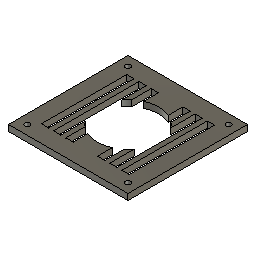
Back Plate (Autodesk Fusion 360 design; units mm, degrees)
part number: 2026-08-30-01-23-59-414
Autodesk Fusion 360 part; units mm, degrees
sketch "Sketch1" plane through (0, 0, 0) normal (0, 0, 1) x (1, 0, 0)
  line L0 (0, 0) -> (98, 0)
  line L1 (98, 0) -> (98, 98)
  line L2 (98, 98) -> (0, 98)
  line L3 (0, 98) -> (0, 0)
extrude "Extrude1" add sketch "Sketch1" along normal blind 5
sketch "Sketch2" plane through (0, 0, 0) normal (0, 0, 1) x (1, 0, 0)
  circle A0 centre (7.75, 7.75) radius 2.1
extrude "Extrude2" cut sketch "Sketch2" along normal blind 5
sketch "Sketch3" plane through (0, 0, 0) normal (0, 0, 1) x (1, 0, 0)
  circle A0 centre (7.75, 90.25) radius 2.1
extrude "Extrude3" cut sketch "Sketch3" along normal blind 5
sketch "Sketch4" plane through (0, 0, 0) normal (0, 0, 1) x (1, 0, 0)
  circle A0 centre (90.25, 7.75) radius 2.1
extrude "Extrude4" cut sketch "Sketch4" along normal blind 5
sketch "Sketch5" plane through (0, 0, 0) normal (0, 0, 1) x (1, 0, 0)
  circle A0 centre (90.25, 90.25) radius 2.1
extrude "Extrude5" cut sketch "Sketch5" along normal blind 5
sketch "Sketch6" plane through (0, 0, 0) normal (0, 0, 1) x (1, 0, 0)
  circle A0 centre (49, 49) radius 25
extrude "Extrude6" cut sketch "Sketch6" along normal blind 5
sketch "Sketch7" plane through (0, 0, 0) normal (0, 0, 1) x (1, 0, 0)
  line L0 (13, 14) -> (19, 14)
  line L1 (19, 14) -> (19, 84)
  line L2 (19, 84) -> (13, 84)
  line L3 (13, 84) -> (13, 14)
extrude "Extrude7" cut sketch "Sketch7" along normal blind 5
sketch "Sketch8" plane through (0, 0, 0) normal (0, 0, 1) x (1, 0, 0)
  line L0 (23, 14) -> (29, 14)
  line L1 (29, 14) -> (29, 84)
  line L2 (29, 84) -> (23, 84)
  line L3 (23, 84) -> (23, 14)
extrude "Extrude8" cut sketch "Sketch8" along normal blind 5
sketch "Sketch9" plane through (0, 0, 0) normal (0, 0, 1) x (1, 0, 0)
  line L0 (33, 14) -> (39, 14)
  line L1 (39, 14) -> (39, 84)
  line L2 (39, 84) -> (33, 84)
  line L3 (33, 84) -> (33, 14)
extrude "Extrude9" cut sketch "Sketch9" along normal blind 5
sketch "Sketch10" plane through (0, 0, 0) normal (0, 0, 1) x (1, 0, 0)
  line L0 (59, 14) -> (65, 14)
  line L1 (65, 14) -> (65, 84)
  line L2 (65, 84) -> (59, 84)
  line L3 (59, 84) -> (59, 14)
extrude "Extrude10" cut sketch "Sketch10" along normal blind 5
sketch "Sketch11" plane through (0, 0, 0) normal (0, 0, 1) x (1, 0, 0)
  line L0 (69, 14) -> (75, 14)
  line L1 (75, 14) -> (75, 84)
  line L2 (75, 84) -> (69, 84)
  line L3 (69, 84) -> (69, 14)
extrude "Extrude11" cut sketch "Sketch11" along normal blind 5
sketch "Sketch12" plane through (0, 0, 0) normal (0, 0, 1) x (1, 0, 0)
  line L0 (79, 14) -> (85, 14)
  line L1 (85, 14) -> (85, 84)
  line L2 (85, 84) -> (79, 84)
  line L3 (79, 84) -> (79, 14)
extrude "Extrude12" cut sketch "Sketch12" along normal blind 5
